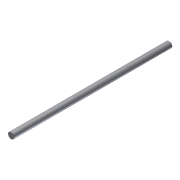
# Autodesk Inventor part: BallShoot Axle
Saved by Autodesk Inventor 2015 SP1 (Build 190203100, 203)
## iProperties
Created: 2014-09-14
Part Number: BallShoot Axle
Document SubType Name: Modeling
Designer: Family Room
Density: 1 g/cm^3
Material: Generic
Appearance: Default
Author: Family Room
Autodesk Inventor part; units mm, degrees
ref_plane "YZ Plane" through (0, 0, 0) normal (1, 0, 0) x (0, 1, 0)
ref_plane "XZ Plane" through (0, 0, 0) normal (0, 1, 0) x (-1, 0, 0)
sketch "Sketch1" plane through (0, 0, 0) normal (0, 0, 1) x (1, 0, 0)
  arc A0 (-1.0878, 2.1) -> (1.0878, 2.1) centre (0, 0) ccw
  line L0 (1.0878, 2.1) -> (-1.0878, 2.1)
  constraints: 2 end point, 2 point on circle, 1 centre point
extrude "Extrusion1" add sketch "Sketch1" along normal blind 120.65
ref_plane "Work Plane1" through (0, 0, 60.325) normal (0, 0, 1) x (1, 0, 0)
body "Solid1"
